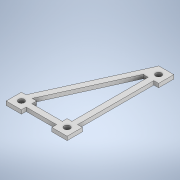
# Autodesk Inventor part: HexServoCoverV2
Saved by Autodesk Inventor 2020 (Build 240168000, 168)
## iProperties
Created: 2023-12-31
Part Number: HexServoCoverV2
Material: Generic
Document SubType Name: Modeling
Designer: smz3rm
Density: 1 g/cm^3
Appearance: Default
Author: smz3rm
Autodesk Inventor part; units mm, degrees
ref_plane "YZ Plane" through (0, 0, 0) normal (1, 0, 0) x (0, 1, 0)
ref_plane "XZ Plane" through (0, 0, 0) normal (0, 1, 0) x (-1, 0, 0)
ref_plane "XY Plane" through (0, 0, 0) normal (0, 0, 1) x (1, 0, 0)
derived "HexBodyV2.ipt"
sketch "Sketch14" plane through (-60, -12, 62.4426) normal (0, 1, 0) x (1, 0, 0)
  line L0 (8, 63.7574) -> (49, 63.7574)
  line L1 (49, 63.7574) -> (49, 23.7574)
  line L2 (49, 23.7574) -> (8, 23.7574)
  line L3 (8, 23.7574) -> (8, 63.7574)
  line L4 (52, 66.7574) -> (4.5, 66.7574)
  line L5 (4.5, 20.7574) -> (52, 20.7574)
  line L6 (52, 20.7574) -> (52, 66.7574)
  line L7 (41, 66.7574) -> (41, 20.7574)
  line L8 (36, 66.7574) -> (36, 20.7574)
  line L9 (8, 63.7574) -> (36, 63.7574)
  line L10 (4, 43.7574) -> (52, 43.7574)
  line L11 (16.5, 66.7574) -> (16.5, 63.7574)
  line L12 (12, 66.7574) -> (12, 63.7574)
  line L13 (49, 53.7574) -> (55, 53.7574)
  line L14 (55, 53.7574) -> (60, 53.7574)
  line L15 (60, 167.4426) -> (60, -42.5574)
  line L16 (49, 68.5926) -> (49, 66.2926)
  line L17 (4.5, 66.7574) -> (4, 66.7574)
  line L18 (4, 8.833) -> (4, 87.1926)
  line L19 (4, 0.833) -> (4, 124.0523)
  line L20 (4.5, 20.7574) -> (4, 20.7574)
  line L21 (36, 23.7574) -> (28, 23.7574)
  line L22 (28, 23.7574) -> (28, 15.7574)
  line L23 (28, 15.7574) -> (36, 15.7574)
  line L24 (36, 15.7574) -> (36, 23.7574)
  line L25 (28, 63.7574) -> (28, 71.7574)
  line L26 (28, 71.7574) -> (36, 71.7574)
  line L27 (36, 71.7574) -> (36, 63.7574)
  line L28 (12, 23.7574) -> (4, 23.7574)
  line L29 (4, 23.7574) -> (4, 15.7574)
  line L30 (4, 15.7574) -> (12, 15.7574)
  line L31 (12, 15.7574) -> (12, 23.7574)
  line L32 (43, 63.8053) -> (43, 88.0017)
  line L33 (43, 66.7574) -> (43, 63.7574)
  line L34 (49, 63.7574) -> (49, 63.8053)
  line L35 (49, 63.8053) -> (43, 63.8053)
  line L36 (49, 63.7574) -> (49, 63.7574)
  line L37 (49, 63.7574) -> (49, 63.8053)
  point P0 (60, 62.4426)
  point P1 (34.5, 20.5208)
  point P2 (41, 65.8053)
  point P3 (49, 67.4426)
  point P4 (49, 43.7574)
  point P5 (41, 23.7574)
  point P6 (28, 66.7574)
  point P7 (36, 20.7574)
  point P8 (28, 20.7574)
  point P9 (12, 20.7574)
  point P10 (41, 63.7574)
sketch "Sketch2" plane through (0, 0, 0) normal (0, 1, 0) x (-1, 0, 0)
  line L0 (32, -1.3148) -> (32, -9.3148) projected
  line L1 (32, -9.3148) -> (24, -9.3148) projected
  line L2 (24, -9.3148) -> (24, -1.3148) projected
  line L3 (32, 38.6852) -> (32, 46.6852) projected
  line L4 (24, 46.6852) -> (24, 38.6852) projected
  line L5 (32, 46.6852) -> (24, 46.6852) projected
  line L6 (56, 46.6852) -> (48, 46.6852) projected
  line L7 (48, 46.6852) -> (48, 38.6852) projected
  line L8 (48, 38.6852) -> (56, 38.6852) projected
  line L9 (56, 38.6852) -> (56, 46.6852)
  line L10 (32, 38.6852) -> (24, 38.6852)
  line L11 (32, -1.3148) -> (24, -1.3148)
  line L12 (32, -9.3148) -> (24, -1.3148)
  line L13 (32, 38.6852) -> (24, 46.6852)
  line L14 (56, 38.6852) -> (48, 46.6852)
  circle A0 centre (28, -5.3148) radius 1.55
  circle A1 centre (28, 42.6852) radius 1.55
  circle A2 centre (52, 42.6852) radius 1.55
  line L15 (48, 41.1852) -> (32, 41.1852)
  line L16 (32, 41.1852) -> (32, 44.1852)
  line L17 (32, 44.1852) -> (48, 44.1852)
  line L18 (48, 44.1852) -> (48, 41.1852)
  line L19 (29.5, -1.3148) -> (26.5, -1.3148)
  line L20 (26.5, -1.3148) -> (26.5, 38.6852)
  line L21 (26.5, 38.6852) -> (29.5, 38.6852)
  line L22 (29.5, 38.6852) -> (29.5, -1.3148)
  line L23 (52, 38.6852) -> (32, -5.3148)
  line L24 (32, -8.9397) -> (53.6477, 38.6852)
  line L25 (29.2689, -7.6983) -> (50.9166, 39.9266)
  point P0 (0, 0)
  point P1 (32, 42.6852)
  point P2 (48, 42.6852)
  point P3 (28, 38.6852)
  point P4 (50.3523, 38.6852)
  point P5 (32, -1.6899)
  point P6 (29.5, 38.6852)
  point P7 (26.5, 38.6852)
  point P8 (26.5, -1.3148)
  dimension "d1" = 3.1
  dimension "d2" = 3.1
  dimension "d3" = 3.1
  dimension "d4" = 3
  dimension "d5" = 3
  dimension "d6" = 3
  constraints: 34 end point, 11 midpoint, 8 parallel, 4 perpendicular, 4 point on line, 3 centre point, 2 horizontal, 2 symmetric about line
  measures "d1" diameter of A0
  measures "d2" diameter of A1
  measures "d3" diameter of A2
  measures "d4" distance between parallel lines of L17 L15
  measures "d5" distance between parallel lines of L20 L22
  measures "d6" distance between parallel lines of L25 L24
extrude "Extrusion1" add sketch "Sketch2" along normal blind 2 contours L23 L8 L24 L0 | L0 L12 L25 | L0 L25 L8 L23 | L25 L12 A0 L11 L0 | L8 L7 L14 A2 | L1 L2 L12 A0 | L14 A2 L6 L9 | L11 L20 L10 L22 | L10 L4 L13 A1 | L15 L3 L17 L7 | L13 A1 L5 L3
equation "\"d1\" = M3ScrewDia"
equation "\"d2\" = M3ScrewDia"
equation "\"d3\" = M3ScrewDia"
equation "\"d5\" = d4"
equation "\"d6\" = d5"
equation "\"M3ScrewDia\" = 3.1"
body "Solid1"
